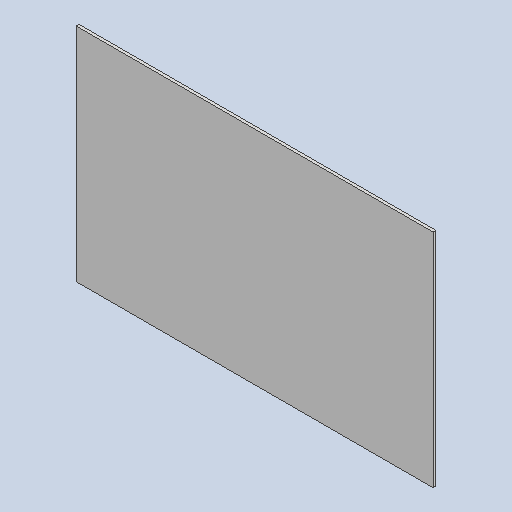
# Autodesk Inventor part: FP-C0603C-CF-IPC_B_CMP-001-00126-1
Saved by Autodesk Inventor 2024.3 (Build 283343000, 343)
## iProperties
Created: 2024-08-24
Part Number: FP-C0603C-CF-IPC_B_CMP-001-00126-1
Material: Generic
Document SubType Name: Modeling
Designer: atrus
Density: 1 g/cm^3
Appearance: Default
Author: atrus
Autodesk Inventor part; units mm, degrees
ref_plane "YZ Plane" through (0, 0, 0) normal (1, 0, 0) x (0, 1, 0)
ref_plane "XZ Plane" through (0, 0, 0) normal (0, 1, 0) x (-1, 0, 0)
ref_plane "XY Plane" through (0, 0, 0) normal (0, 0, 1) x (1, 0, 0)
sketch "Sketch1" plane through (0, 0, 0) normal (0, 0, 1) x (1, 0, 0)
  line L0 (-1.5791, -0.9791) -> (1.5791, -0.9791)
  line L1 (1.5791, -0.9791) -> (1.5791, 0.9791)
  line L2 (1.5791, 0.9791) -> (-1.5791, 0.9791)
  line L3 (-1.5791, 0.9791) -> (-1.5791, -0.9791)
  constraints: 8 end point
extrude "Extrusion1" add sketch "Sketch1" along normal blind 0.0254
body "Solid1"
